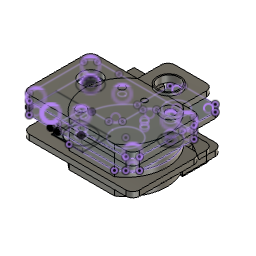
Gearbox v15 (Autodesk Fusion 360 design; units mm, degrees)
Autodesk Fusion 360 part; units mm, degrees
note: some values were not read from the file. Chosen so that the rebuilt part matches the saved one: which face or edge a step refers to; which pieces of a blend or face edit are solid. Set by a fixed rule: which sketch regions a step uses.
sketch "Sketch1" plane through (0, 0, 0) normal (0, 0, 1) x (1, 0, 0) in component "Version 1 Bottom"
  line L0 (5, 5) -> (-6, 5)
  line L1 (-6, 5) -> (-6, -5) construction
  line L2 (-6, -5) -> (5, -5)
  line L3 (6, -4) -> (6, 4)
  line L4 (6, 5) -> (-6, -5) construction
  line L5 (-6, 5) -> (6, -5) construction
  circle A0 centre (3.5799, 2.9833) radius 0.675
  circle A1 centre (-3.5799, -2.9833) radius 0.675
  circle A2 centre (0, 0) radius 1.975
  circle A3 centre (0, 2.735) radius 0.4
  line L6 (0, 1.75) -> (0, 22.5)
  circle A4 centre (-3.2599, 2.7166) radius 0.45
  line L7 (-6, 5) -> (-9.1769, 5)
  line L8 (-10.1769, 4) -> (-10.1769, -4)
  line L9 (-9.1769, -5) -> (-6, -5)
  circle A5 centre (-6.7769, 1.6) radius 0.46
  line L10 (-3.2599, 2.7166) -> (-6.7769, 1.6) construction
  arc A6 (-9.1769, 5) -> (-10.1769, 4) centre (-9.1769, 4) ccw
  arc A7 (-10.1769, -4) -> (-9.1769, -5) centre (-9.1769, -4) ccw
  arc A8 (5, -5) -> (6, -4) centre (5, -4) ccw
  arc A9 (6, 4) -> (5, 5) centre (5, 4) ccw
  circle A10 centre (-6.7769, 1.6) radius 3.4 construction
  circle A11 centre (-3.5799, -2.9833) radius 1.675 construction
  point P0 (-10.1769, -5)
  dimension "d9" = 10
  dimension "d10" = 12
  dimension "d12" = 1.35
  dimension "d13" = 1.35
  dimension "d15" = 3.95
  dimension "d16" = 0.8
  dimension "d18" = 0.9
  dimension "d19" = 3.26
  dimension "d22" = 2.735
  dimension "d27" = 9.32
  dimension "d28" = 4.66
  dimension "d29" = 0.92
  dimension "d31" = 3.69
  dimension "d32" = 1
  dimension "d33" = 1
  dimension "d34" = 1
  dimension "d57" = 6.8
  dimension "d58" = 3.35
  constraint horizontal L0
  constraint perpendicular L0 L1
  constraint parallel L0 L2
  constraint parallel L1 L3
  constraint coincident L4 A2.centre
  constraint coincident L5 A2.centre
  constraint coincident A2.centre origin
  constraint coincident L4 A0.centre
  constraint coincident L4 A1.centre
  constraint coincident A3.centre L6
  constraint coincident L5 A4.centre
  constraint horizontal L7
  constraint vertical L8
  constraint horizontal L9
  constraint collinear L2 L9
  constraint coincident A4.centre L10.start
  constraint coincident A5.centre L10.end
  constraint coincident L1.end L2.start
  constraint tangent L7 A6
  constraint tangent L8 A6
  constraint coincident P0 L8
  constraint coincident P0 L9
  constraint tangent L8 A7
  constraint tangent L9 A7
  constraint equal A6 A7
  constraint coincident L5.end L2
  constraint coincident L5.end L3
  constraint tangent L2 A8
  constraint tangent L3 A8
  constraint coincident L4.start L0
  constraint coincident L4.start L3
  constraint tangent L0 A9
  constraint tangent L3 A9
  constraint concentric A5 A10
  constraint concentric A1 A11
  constraint tangent L0 A10
  constraint tangent L8 A10
  measures "d9" distance of L4.start L5.end
  measures "d10" distance of L4.start L0.end
  measures "d12" diameter of A0
  measures "d13" diameter of A1
  measures "d15" diameter of A2
  measures "d16" diameter of A3
  measures "d18" diameter of A4
  measures "d19" distance of A3.centre A4.centre
  measures "d22" distance of A2.centre A3.centre
  measures "d27" distance of A0.centre A1.centre
  measures "d28" distance of A1.centre A2.centre
  measures "d29" diameter of A5
  measures "d31" distance of A4.centre A5.centre
  measures "d32" radius of A6
  measures "d33" radius of A8
  measures "d34" radius of A9
  measures "d57" diameter of A10
  measures "d58" diameter of A11
extrude "Extrude1" add sketch "Sketch1" along normal blind 0.8 makes body 1 in component "Version 1 Bottom"
ref_plane "WorkPlane1" through (-2.0885, 0, 3.25) normal (0, 0, 1) x (1, 0, 0) in component "Layer2"
sketch "Sketch1 (2)" plane through (0, 0, 3.25) normal (0, 0, 1) x (1, 0, 0) in component "Layer2"
  circle A0 centre (3.5799, 2.9833) radius 0.675
  circle A1 centre (-3.5799, -2.9833) radius 0.675
  line L0 (5, 5) -> (-0.5, 5)
  line L1 (-6, -1) -> (-6, -4)
  line L2 (-5, -5) -> (5, -5)
  line L3 (6, -4) -> (6, 4)
  line L4 (6, 5) -> (-6, -5) construction
  line L5 (-6, 5) -> (6, -5) construction
  circle A2 centre (0, 2.735) radius 0.4
  line L6 (-6, 5) -> (-1.5, 5)
  line L7 (-1.5, 4) -> (-1.5, 1)
  line L8 (-2.5, 0) -> (-5, 0)
  line L9 (-6, 0) -> (-6, 5)
  circle A3 centre (-3.5799, -2.9833) radius 0.675
  arc A4 (-6, -4) -> (-5, -5) centre (-5, -4) ccw
  arc A5 (-5, 0) -> (-6, -1) centre (-5, -1) ccw
  arc A6 (-2.5, 0) -> (-1.5, 1) centre (-2.5, 1) ccw
  arc A7 (-0.5, 5) -> (-1.5, 4) centre (-0.5, 4) ccw
  arc A8 (6, 4) -> (5, 5) centre (5, 4) ccw
  arc A9 (5, -5) -> (6, -4) centre (5, -4) ccw
  dimension "d40" = 10
  dimension "d41" = 12
  dimension "d43" = 1.5
  dimension "d44" = 1
  dimension "d45" = 1
  dimension "d46" = 1
  dimension "d47" = 1
  dimension "d48" = 1
  dimension "d49" = 1
  constraint horizontal L0
  constraint perpendicular L0 L1
  constraint parallel L0 L2
  constraint parallel L1 L3
  constraint coincident L4 origin
  constraint coincident L5 origin
  constraint horizontal L6
  constraint vertical L7
  constraint horizontal L8
  constraint vertical L9
  constraint coincident origin L8
  constraint coincident L4.end L2
  constraint coincident L4.end L1
  constraint tangent L2 A4
  constraint tangent L1 A4
  constraint coincident L9.start L8
  constraint coincident L5.start L1
  constraint tangent L8 A5
  constraint tangent L1 A5
  constraint tangent L7 A6
  constraint tangent L8 A6
  constraint coincident L6.end L7
  constraint coincident L5.start L0
  constraint tangent L7 A7
  constraint tangent L0 A7
  constraint coincident L4.start L3
  constraint coincident L4.start L0
  constraint tangent L3 A8
  constraint tangent L0 A8
  constraint coincident L5.end L3
  constraint coincident L5.end L2
  constraint tangent L3 A9
  constraint tangent L2 A9
  measures "d40" distance of L4.start L5.end
  measures "d41" distance of L1 L3
  measures "d43" distance of A2.centre L7
  measures "d44" radius of A4
  measures "d45" radius of A5
  measures "d46" radius of A6
  measures "d47" radius of A7
  measures "d48" radius of A8
  measures "d49" radius of A9
extrude "Extrude1'" add sketch "Sketch1 (2)" along normal blind 0.8 separate body makes body 2 in component "Layer2"
ref_plane "WorkPlane1" through (-2.0885, 0, 5.02) normal (0, 0, 1) x (1, 0, 0) in component "Layer3"
sketch "Sketch1 (3)" plane through (0, 0, 5.02) normal (0, 0, 1) x (1, 0, 0) in component "Layer3"
  circle A0 centre (3.5799, 2.9833) radius 0.675
  circle A1 centre (-3.5799, -2.9833) radius 0.675
  circle A2 centre (-6.7769, 1.6) radius 0.46
  circle A3 centre (-3.2599, 2.7166) radius 0.45
  circle A4 centre (-6.7769, 1.6) radius 1.52
  arc A5 (-9.1769, 5) -> (-10.1769, 4) centre (-9.1769, 4) ccw
  line L0 (-10.1769, 4) -> (-10.1769, -4)
  arc A6 (-10.1769, -4) -> (-9.1769, -5) centre (-9.1769, -4) ccw
  line L1 (-9.1769, -5) -> (-6, -5)
  line L2 (-6, -5) -> (5, -5)
  arc A7 (5, -5) -> (6, -4) centre (5, -4) ccw
  line L3 (6, -4) -> (6, 4)
  arc A8 (6, 4) -> (5, 5) centre (5, 4) ccw
  line L4 (5, 5) -> (-6, 5)
  line L5 (-6, 5) -> (-9.1769, 5)
  dimension "d55" = 3.04
  constraint concentric A2 A4
  measures "d55" diameter of A4
extrude "Extrude1''" add sketch "Sketch1 (3)" along normal blind 0.8 separate body contours A5 L0 A6 L1 L2 A7 L3 A8 L4 L5 makes body 3 in component "Layer3"
sketch "Sketch1 (4)" plane through (0, 0, 3.25) normal (0, 0, -1) x (1, 0, 0) in component "Version 1 Upper"
  circle A0 centre (0, -2.735) radius 0.4
  circle A1 centre (-3.5799, 2.9833) radius 0.675
  circle A2 centre (3.5799, -2.9833) radius 0.675
  line L0 (-5, 0) -> (-2.5, 0)
  arc A3 (-1.5, -1) -> (-2.5, 0) centre (-2.5, -1) ccw
  line L1 (-1.5, -1) -> (-1.5, -4)
  arc A4 (-1.5, -4) -> (-0.5, -5) centre (-0.5, -4) ccw
  line L2 (-0.5, -5) -> (5, -5)
  arc A5 (5, -5) -> (6, -4) centre (5, -4) ccw
  line L3 (6, -4) -> (6, 4)
  arc A6 (6, 4) -> (5, 5) centre (5, 4) ccw
  line L4 (5, 5) -> (-5, 5)
  arc A7 (-5, 5) -> (-6, 4) centre (-5, 4) ccw
  line L5 (-6, 4) -> (-6, 1)
  arc A8 (-6, 1) -> (-5, 0) centre (-5, 1) ccw
  line L6 (-10.1769, -4) -> (-10.1769, 4)
  arc A9 (-9.1769, 5) -> (-10.1769, 4) centre (-9.1769, 4) ccw
  line L7 (-9.1769, 5) -> (-6, 5)
  line L8 (-6, 5) -> (-5, 5)
  line L9 (-5, 0) -> (-10.1769, 0)
  line L10 (-10.1769, 0) -> (-10.1769, 4)
  constraint coincident L7.end L8.start
  constraint coincident L4.end A7.start
  constraint coincident L0.start A8.end
  constraint coincident L6.end A9.end
  constraint midpoint L6 L9.end
sketch "Sketch2" plane through (0, 0, 5.02) normal (0, 0, -1) x (1, 0, 0) in component "Version 1 Upper"
  circle A0 centre (-6.7769, -1.6) radius 1.52
  circle A1 centre (-3.2599, -2.7166) radius 0.45
  circle A2 centre (3.5799, -2.9833) radius 0.675
  circle A3 centre (-3.5799, 2.9833) radius 0.675
  line L0 (-9.1769, -5) -> (5, -5)
  arc A4 (5, -5) -> (6, -4) centre (5, -4) ccw
  line L1 (6, -4) -> (6, 4)
  arc A5 (6, 4) -> (5, 5) centre (5, 4) ccw
  line L2 (5, 5) -> (-9.1769, 5)
  arc A6 (-9.1769, 5) -> (-10.1769, 4) centre (-9.1769, 4) ccw
  line L3 (-10.1769, 4) -> (-10.1769, -4)
  arc A7 (-10.1769, -4) -> (-9.1769, -5) centre (-9.1769, -4) ccw
  circle A8 centre (-3.2599, -2.7166) radius 0.9
  circle A9 centre (-6.7769, -1.6) radius 3.025
  circle A10 centre (-3.2599, -2.7166) radius 0.65
  circle A11 centre (-6.7769, -1.6) radius 1.72
  dimension "d147" = 1.8
  dimension "d148" = 6.05
  dimension "d152" = 0.2
  dimension "d155" = 0.2
  constraint concentric A1 A8
  constraint concentric A0 A9
  constraint concentric A1 A10
  constraint concentric A0 A11
  measures "d147" diameter of A8
  measures "d148" diameter of A9
  measures "d152" distance of A1 A10
  measures "d155" distance of A0 A11
extrude "Extrude1'''" add sketch "Sketch2" against normal blind 0.8 separate body contours L0 A4 L1 A5 L2 A6 L3 A7 | A8 A9 | A8 A9 | A8 A9 | A10 | A11 makes body 4 in component "Version 1 Upper"
extrude "Extrude2" add sketch "Sketch1 (4)" against normal up to surface (1.77 mm away) bodies 4 in component "Version 1 Upper"
sketch "Sketch1 (5)" plane through (0, 0, 0) normal (0, 0, 1) x (1, 0, 0) in component "Calibration"
  circle A0 centre (-3.5799, -2.9833) radius 0.675
  circle A1 centre (-3.2599, 2.7166) radius 0.45
  circle A2 centre (-6.7769, 1.6) radius 0.46
  circle A3 centre (0, 2.735) radius 0.4
  circle A4 centre (3.5799, 2.9833) radius 0.675
  circle A5 centre (0, 0) radius 1.975
  arc A6 (6, 4) -> (5, 5) centre (5, 4) ccw
  line L0 (5, 5) -> (-9.1769, 5)
  arc A7 (-9.1769, 5) -> (-10.1769, 4) centre (-9.1769, 4) ccw
  line L1 (-10.1769, 4) -> (-10.1769, -4)
  arc A8 (-10.1769, -4) -> (-9.1769, -5) centre (-9.1769, -4) ccw
  line L2 (-9.1769, -5) -> (5, -5)
  arc A9 (5, -5) -> (6, -4) centre (5, -4) ccw
  line L3 (6, -4) -> (6, 4)
  circle A10 centre (-6.6616, -1.798) radius 1.52
  circle A11 centre (-6.7769, 1.6) radius 3.4
  dimension "d68" = 3.04
  dimension "d70" = 6.9
  constraint coincident A10.centre A11
  measures "d68" diameter of A10
  measures "d70" distance of A10.centre A5.centre
extrude "Extrude1''''" add sketch "Sketch1 (5)" along normal blind 0.8 separate body contours A1 A6 L0 L1 A8 L2 A9 L3 A10 A11 | A1 A10 A11 | L0 A7 L1 A11 makes body 5 in component "Calibration"
sketch "Sketch1 (6)" plane through (0, 0, 0) normal (0, 0, 1) x (1, 0, 0) in component "Version 2"
  circle A0 centre (0, 0) radius 6
  line L0 (6, 5) -> (-6, 5)
  line L1 (-6, 5) -> (-6, -5) construction
  line L2 (-6, -5) -> (6, -5)
  line L3 (6, -5) -> (6, 5) construction
  line L4 (6, 5) -> (-6, -5) construction
  line L5 (-6, 5) -> (6, -5) construction
  circle A1 centre (0, 0) radius 1.975
  circle A2 centre (3.5799, 2.9833) radius 0.675
  circle A3 centre (-3.5799, -2.9833) radius 0.675
  circle A4 centre (0, 2.735) radius 0.4
  line L6 (0, 1.75) -> (0, 22.5)
  line L7 (-3.3166, 5) -> (3.3166, 5)
  line L8 (-3.3166, 5) -> (3.3166, 5)
  line L9 (3.3166, 5) -> (3.3166, 6.4944)
  line L10 (3.311, 6.5) -> (-3.3116, 6.5)
  line L11 (-3.3166, 6.495) -> (-3.3166, 5)
  arc A5 (3.3166, 6.4944) -> (3.311, 6.5) centre (3.311, 6.4944) ccw
  arc A6 (-3.3116, 6.5) -> (-3.3166, 6.495) centre (-3.3116, 6.495) ccw
  dimension "d73" = 12
  dimension "d74" = 10
  dimension "d75" = 12
  dimension "d76" = 3.95
  dimension "d100" = 1.5
  constraint coincident A0.centre A1.centre
  constraint horizontal L0
  constraint perpendicular L0 L1
  constraint parallel L0 L2
  constraint parallel L1 L3
  constraint coincident L4 A0.centre
  constraint coincident L5 A0.centre
  constraint horizontal L7
  constraint coincident A0 L7.start
  constraint coincident A0 L7.end
  constraint coincident L0 L7.start
  constraint horizontal L8
  constraint vertical L9
  constraint horizontal L10
  constraint vertical L11
  constraint coincident L7.end L8.end
  constraint tangent L9 A5
  constraint tangent L10 A5
  constraint tangent L10 A6
  constraint tangent L11 A6
  measures "d73" diameter of A0
  measures "d74" distance of L0.start L2.end
  measures "d75" distance of L1.end L2.end
  measures "d76" diameter of A1
  measures "d100" distance of L8 L10
extrude "Extrude1'''''" add sketch "Sketch1 (6)" against normal blind 0.8 separate body contours A0 L0 L2 L7 L8 | A0 L0 L6 L7 L8 | A0 L6 L9 L10 A5 | A0 L0 L6 L7 L8 | A0 L6 L10 L11 A6 makes body 6 in component "Version 2"
ref_plane "WorkPlane1" through (0, 0.75, -2.4) normal (0, 0, 1) x (1, 0, 0) in component "Version 2"
sketch "Sketch2 (2)" plane through (0, 0, -2.4) normal (0, 0, 1) x (1, 0, 0) in component "Version 2"
  circle A0 centre (0, 7.42) radius 0.46
  line L0 (0, 1.75) -> (0, 22.5)
  circle A1 centre (0, 2.735) radius 0.4
  circle A2 centre (0, 0) radius 6
  line L1 (-3.3166, 5) -> (3.3166, 5)
  line L2 (-3.3166, 5) -> (3.3166, 5)
  line L3 (3.3166, 5) -> (3.3166, 9.8)
  line L4 (2.3166, 10.8) -> (-2.3166, 10.8)
  line L5 (-3.3166, 9.8) -> (-3.3166, 5)
  arc A3 (-2.3166, 10.8) -> (-3.3166, 9.8) centre (-2.3166, 9.8) ccw
  arc A4 (3.3166, 9.8) -> (2.3166, 10.8) centre (2.3166, 9.8) ccw
  circle A5 centre (0, 7.42) radius 1
  point P0 (3.3166, 10.8)
  point P1 (3.3166, 5)
  dimension "d88" = 0.92
  dimension "d89" = 4.685
  dimension "d90" = 5.8
  dimension "d91" = 1
  dimension "d92" = 1
  dimension "d99" = 2
  constraint coincident A0.centre L0
  constraint horizontal L2
  constraint vertical L3
  constraint horizontal L4
  constraint vertical L5
  constraint coincident L1.start L2.start
  constraint coincident P1 L1.end
  constraint tangent L4 A3
  constraint tangent L5 A3
  constraint coincident P0 L3
  constraint coincident P0 L4
  constraint tangent L3 A4
  constraint tangent L4 A4
  constraint concentric A0 A5
  measures "d88" diameter of A0
  measures "d89" distance of A0.centre A1.centre
  measures "d90" distance of P1 P0
  measures "d91" radius of A3
  measures "d92" radius of A4
  measures "d99" diameter of A5
extrude "Extrude2'" add sketch "Sketch2 (2)" against normal blind 0.8 separate body contours A0 L0 A5 | A0 L0 A5 | L0 A2 L4 L5 A3 A5 | L0 A2 L3 L4 A4 A5 | L0 A2 L1 L2 | L0 A2 L1 L2 makes body 7 in component "Version 2"
extrude "Extrude3" add sketch "Sketch1 (6)" against normal up to surface (2.4 mm away) contours A0 L0 L6 L7 L8 | A0 L6 L9 L10 A5 | A0 L0 L6 L7 L8 | A0 L6 L10 L11 A6 bodies 6 7 in component "Version 2"
ref_plane "WorkPlane2" through (0, 0.75, 1.65) normal (0, 0, -1) x (-1, 0, 0) in component "Version 2"
sketch "Sketch1 (7)" plane through (0, 0, 1.65) normal (0, 0, -1) x (-1, 0, 0) in component "Upper Deck"
  arc A0 (-3.3166, 5) -> (-3.3166, -5) centre (0, 0) ccw
  line L0 (-3.3166, -5) -> (3.3166, -5)
  arc A1 (3.3166, -5) -> (3.3166, 5) centre (0, 0) ccw
  circle A2 centre (0, 0) radius 1.975
  circle A3 centre (3.5799, -2.9833) radius 0.675
  circle A4 centre (-3.5799, 2.9833) radius 0.675
  circle A5 centre (0, 2.735) radius 0.4
  line L1 (-3.3166, 6.4944) -> (-3.3166, 9.8)
  arc A6 (-2.3166, 10.8) -> (-3.3166, 9.8) centre (-2.3166, 9.8) ccw
  line L2 (-2.3166, 10.8) -> (2.3166, 10.8)
  arc A7 (3.3166, 9.8) -> (2.3166, 10.8) centre (2.3166, 9.8) ccw
  line L3 (3.3166, 9.8) -> (3.3166, 6.495)
  circle A8 centre (0, 7.42) radius 0.46
  circle A9 centre (0, 7.42) radius 1.52
  line L4 (3.3166, 5) -> (-3.3166, 5)
  line L5 (3.3166, 6.495) -> (3.3166, 5)
  line L6 (-3.3166, 6.4944) -> (-3.3166, 5)
  dimension "d104" = 3.04
  constraint concentric A8 A9
  constraint coincident L3.end L5.start
  constraint coincident A1.end L4.start
  constraint coincident L1.start L6.start
  constraint coincident A0.start L4.end
  measures "d104" diameter of A9
extrude "Extrude1''''''" add sketch "Sketch1 (7)" against normal blind 0.8 separate body contours A0 L0 A1 L4 | L1 A6 L2 A7 L3 L4 L5 L6 makes body 8 in component "Upper Deck"
sketch "Sketch1 (8)" plane through (0, 0, 0) normal (0, 0, 1) x (1, 0, 0) in component "Lower Part"
  circle A0 centre (0, 0) radius 6
  line L0 (6, -5) -> (6, 5)
  line L1 (-6, 5) -> (6, -5)
  line L2 (-6, -5) -> (6, -5)
  line L3 (6, 5) -> (-6, -5)
  circle A1 centre (-3.5799, -2.9833) radius 0.675
  circle A2 centre (3.5799, 2.9833) radius 0.675
  line L4 (3.311, 6.5) -> (-3.3116, 6.5)
  line L5 (3.3166, 5) -> (3.3166, 6.4944)
  arc A3 (3.3166, 6.4944) -> (3.311, 6.5) centre (3.311, 6.4944) ccw
  arc A4 (-3.3116, 6.5) -> (-3.3166, 6.495) centre (-3.3116, 6.495) ccw
  line L6 (-3.3166, 6.495) -> (-3.3166, 5)
  line L7 (-3.3166, 5) -> (3.3166, 5)
  line L8 (6, 5) -> (-6, 5)
  line L9 (-6, 5) -> (-6, -5)
  circle A5 centre (0, 2.735) radius 0.4
  point P0 (3.311, 6.4944)
  point P1 (-3.3116, 6.495)
  point P2 (0, 2.735)
  point P3 (0, 1.75)
  point P4 (3.5799, 2.9833)
  point P5 (-3.5799, -2.9833)
extrude "Extrude1'''''''" add sketch "Sketch1 (8)" against normal blind 0.8 separate body contours A0 L7 L8 | A0 L4 L5 A3 A4 L6 | A0 L1 L3 A2 L7 L8 | A0 L1 L3 A2 | A0 L1 L3 A1 | A0 L1 L2 L3 A1 makes body 9 in component "Lower Part"
ref_plane "WorkPlane2" through (0, 0, -1.74) normal (0, 0, 1) x (1, 0, 0) in component "Lower Part"
sketch "Sketch2 (3)" plane through (0, 0, -1.74) normal (0, 0, 1) x (-1, 0, 0) in component "Lower Part"
  arc A0 (-3.3166, -6) -> (-2.8166, -6.5) centre (-2.8166, -6) ccw
  arc A1 (2.8166, -6.5) -> (3.3166, -6) centre (2.8166, -6) ccw
  line L0 (2.8166, -6.5) -> (-2.8166, -6.5)
  circle A2 centre (0, -7.42) radius 0.435
  line L1 (3.3166, -5) -> (-3.3166, -5)
  circle A3 centre (0, -6.305) radius 0.46
  circle A4 centre (0, -2.735) radius 0.38
  circle A5 centre (0, -6.305) radius 0.8
  line L2 (0, -1.75) -> (0, -22.5)
  line L3 (3.3166, -5) -> (-3.3166, -5)
  line L4 (-3.3166, -5) -> (-3.3166, -8.5)
  line L5 (-2.3166, -9.5) -> (2.3166, -9.5)
  line L6 (3.3166, -8.5) -> (3.3166, -5)
  arc A6 (2.3166, -9.5) -> (3.3166, -8.5) centre (2.3166, -8.5) ccw
  arc A7 (-3.3166, -8.5) -> (-2.3166, -9.5) centre (-2.3166, -8.5) ccw
  point P0 (3.3166, -9.5)
  dimension "d109" = 0.92
  dimension "d111" = 3.57
  dimension "d112" = 1.6
  dimension "d113" = 4.5
  dimension "d114" = 1
  dimension "d115" = 1
  constraint concentric A3 A5
  constraint coincident A3.centre L2
  constraint horizontal L3
  constraint vertical L4
  constraint horizontal L5
  constraint vertical L6
  constraint coincident L1.start L3.start
  constraint coincident L1.end L3.end
  constraint coincident P0 L5
  constraint coincident P0 L6
  constraint tangent L5 A6
  constraint tangent L6 A6
  constraint tangent L4 A7
  constraint tangent L5 A7
  measures "d109" diameter of A3
  measures "d111" distance of A3.centre A4.centre
  measures "d112" diameter of A5
  measures "d113" distance of L1.start P0
  measures "d114" radius of A6
  measures "d115" radius of A7
extrude "Extrude2''" add sketch "Sketch2 (3)" against normal blind 1.6 separate body contours A0 L0 L1 A5 L2 L3 L4 | A0 L0 A2 A5 L2 L4 L5 A7 | L0 A3 A5 L2 | L0 A2 A3 A5 L2 | A1 L0 L1 A5 L2 L3 L6 | L0 A3 A5 L2 | A2 A5 L2 | A2 A5 L2 | A1 L0 A2 A5 L2 L5 L6 A6 | L0 A2 A3 A5 L2 | A2 A5 L2 | A2 A5 L2 makes body 10 in component "Lower Part"
extrude "Extrude3'" add sketch "Sketch1 (8)" against normal up to surface (1.74 mm away) contours A0 L7 L8 | A0 L4 L5 A3 A4 L6 bodies 9 10 in component "Lower Part"
extrude "Extrude4" cut sketch "Sketch2 (3)" along normal up to surface (1.74 mm away) contours L0 A3 A5 L2 | L0 A2 A3 A5 L2 | L0 A3 L2 | L0 A3 L2 | L0 A3 A5 L2 | A2 A5 L2 | A2 A5 L2 | L0 A3 L2 | L0 A3 L2 | L0 A2 A3 A5 L2 picked at (-0.1534, -7.2818) picked at (-0.0461, -7.0646) bodies 9 in component "Lower Part"
ref_plane "WorkPlane1" through (0, 0.75, 5) normal (0, 0, 1) x (1, 0, 0) in component "Upper Level"
sketch "Sketch1 (9)" plane through (0, 0, 5) normal (0, 0, 1) x (1, 0, 0) in component "Upper Level"
  line L0 (3.3166, 6.4944) -> (3.3166, 8.5)
  arc A0 (3.3166, 8.5) -> (2.3166, 9.5) centre (2.3166, 8.5) ccw
  line L1 (2.3166, 9.5) -> (-2.3166, 9.5)
  arc A1 (-2.3166, 9.5) -> (-3.3166, 8.5) centre (-2.3166, 8.5) ccw
  line L2 (-3.3166, 8.5) -> (-3.3166, 6.495)
  line L3 (-3.3166, 6.495) -> (-3.3166, 5)
  arc A2 (-3.3166, 5) -> (-3.3166, -5) centre (0, 0) ccw
  line L4 (-3.3166, -5) -> (3.3166, -5)
  arc A3 (3.3166, -5) -> (3.3166, 5) centre (0, 0) ccw
  line L5 (3.3166, 5) -> (3.3166, 6.4944)
  circle A4 centre (3.5799, 2.9833) radius 0.675
  circle A5 centre (0, 2.735) radius 0.4
  circle A6 centre (-3.5799, -2.9833) radius 0.675
  circle A7 centre (0, 6.305) radius 1.52
  point P0 (0, 6.305)
  dimension "d126" = 3.04
  constraint coincident P0 A7.centre
  measures "d126" diameter of A7
extrude "Extrude1''''''''" add sketch "Sketch1 (9)" along normal blind 0.8 separate body makes body 11 in component "Upper Level"
sketch "Sketch5" plane through (3.3166, 0, 0) normal (1, 0, 0) x (0, 1, 0) in component "Version 2"
  line L0 (6.4944, 0) -> (5, 0)
  line L1 (5, 0) -> (5, -0.8)
  line L2 (5, -0.8) -> (5, -3.2)
  line L3 (5, -3.2) -> (9.8, -3.2)
  line L4 (9.8, -3.2) -> (9.8, -2.4)
  line L5 (9.8, -2.4) -> (6.4944, -2.4)
  line L6 (6.4944, -2.4) -> (6.4944, 0)
  line L7 (6.4944, 0) -> (7.42, -2.4)
  line L8 (6.4944, -2.4) -> (6.4944, 0)
  point P0 (7.42, -2.4)
  constraint coincident L0.start L6.end
  constraint coincident P0 L7.end
  constraint coincident L5.end L6.start
extrude "Extrude6" add sketch "Sketch5" against normal up to surface (6.6332 mm away) contours L5 L6 L7 L8 bodies 6 in component "Version 2"
extrude "Extrude7" cut sketch "Sketch2 (2)" along normal up to surface (2.4 mm away) contours A0 L0 | A0 L0 A5 | A0 L0 | A0 L0 A5 bodies 6 in component "Version 2"
sketch "Sketch2 (4)" plane through (0, 0, 5.8) normal (0, 0, 1) x (-1, 0, 0) in component "Upper Level"
  circle A0 centre (0, -6.305) radius 1.52
  circle A1 centre (-3.5799, -2.9833) radius 0.675
  circle A2 centre (0, -2.735) radius 0.4
  circle A3 centre (3.5799, 2.9833) radius 0.675
  line L0 (-3.3166, -5) -> (-3.3166, -8.5)
  arc A4 (-3.3166, -8.5) -> (-2.3166, -9.5) centre (-2.3166, -8.5) ccw
  line L1 (-2.3166, -9.5) -> (2.3166, -9.5)
  arc A5 (2.3166, -9.5) -> (3.3166, -8.5) centre (2.3166, -8.5) ccw
  line L2 (3.3166, -8.5) -> (3.3166, -5)
  arc A6 (3.3166, -5) -> (3.3166, 5) centre (0, 0) ccw
  line L3 (3.3166, 5) -> (-3.3166, 5)
  arc A7 (-3.3166, 5) -> (-3.3166, -5) centre (0, 0) ccw
  circle A8 centre (0, -6.305) radius 1.52
  circle A9 centre (0, -6.305) radius 1.72
  dimension "d140" = 0.2
  constraint concentric A8 A9
  measures "d140" distance of A8 A9
extrude "Extrude2'''" add sketch "Sketch2 (4)" along normal blind 0.4 contours A9 bodies 11 in component "Upper Level"
sketch "Sketch3" plane through (0, 0, 5) normal (0, 0, -1) x (1, 0, 0) in component "Upper Level"
  circle A0 centre (0, -6.305) radius 1.52
  circle A1 centre (3.5799, -2.9833) radius 0.675
  circle A2 centre (0, -2.735) radius 0.4
  circle A3 centre (-3.5799, 2.9833) radius 0.675
  line L0 (3.3166, -8.5) -> (3.3166, -5)
  arc A4 (3.3166, -5) -> (3.3166, 5) centre (0, 0) ccw
  line L1 (3.3166, 5) -> (-3.3166, 5)
  arc A5 (-3.3166, 5) -> (-3.3166, -5) centre (0, 0) ccw
  line L2 (-3.3166, -5) -> (-3.3166, -8.5)
  arc A6 (-3.3166, -8.5) -> (-2.3166, -9.5) centre (-2.3166, -8.5) ccw
  line L3 (-2.3166, -9.5) -> (2.3166, -9.5)
  arc A7 (2.3166, -9.5) -> (3.3166, -8.5) centre (2.3166, -8.5) ccw
  circle A8 centre (0, -6.305) radius 3.025
  point P0 (0, -6.305)
  dimension "d143" = 6.05
  constraint coincident P0 A0.centre
  measures "d143" diameter of A8
extrude "Extrude3''" cut sketch "Sketch3" against normal blind 0.2 contours A8 bodies 11 in component "Upper Level"
extrude "Extrude3'''" cut sketch "Sketch2" along normal through all contours A8 A9 | A11 picked at (-4.6148, -2.9553) bodies 4 in component "Version 1 Upper"
extrude "Extrude4'" add sketch "Sketch2" along normal blind 0.2 contours A10 bodies 4 in component "Version 1 Upper"
extrude "Extrude5" add sketch "Sketch2" along normal blind 0.2 contours A11 bodies 4 in component "Version 1 Upper"
extrude "Extrude6'" cut sketch "Sketch1 (4)" against normal up to surface (2.57 mm away) contours A0 bodies 4 in component "Version 1 Upper"
fillet "Fillet3" radius 1 3 edges at (-4.2097, 0, 4.135) (-9.3442, 0, 4.135) (-10.1769, 0, 4.135) on bodies 4 in component "Version 1 Upper"
sketch "Sketch2 (5)" plane through (0, 0, 1.65) normal (0, 0, -1) x (1, 0, 0) in component "Upper Deck"
  circle A0 centre (0, -7.42) radius 1.52
  circle A1 centre (0, 0) radius 1.975
  circle A2 centre (0, -2.735) radius 0.4
  circle A3 centre (-3.5799, 2.9833) radius 0.675
  circle A4 centre (3.5799, -2.9833) radius 0.675
  arc A5 (2.3166, -10.8) -> (3.3166, -9.8) centre (2.3166, -9.8) ccw
  line L0 (3.3166, -9.8) -> (3.3166, -5)
  arc A6 (3.3166, -5) -> (3.3166, 5) centre (0, 0) ccw
  line L1 (3.3166, 5) -> (-3.3166, 5)
  arc A7 (-3.3166, 5) -> (-3.3166, -5) centre (0, 0) ccw
  line L2 (-3.3166, -5) -> (-3.3166, -9.8)
  arc A8 (-3.3166, -9.8) -> (-2.3166, -10.8) centre (-2.3166, -9.8) ccw
  line L3 (-2.3166, -10.8) -> (2.3166, -10.8)
  circle A9 centre (0, -7.42) radius 2.52
  dimension "d166" = 1
  constraint concentric A0 A9
  measures "d166" distance of A0 A9
extrude "Extrude3''''" add sketch "Sketch2 (5)" along normal blind 0.8 contours A9 bodies 8 in component "Upper Deck"
sketch "Sketch1 (10)" plane through (0, 0, 2.45) normal (0, 0, 1) x (-1, 0, 0) in component "Distancers"
  circle A0 centre (0, -7.42) radius 1.52
  circle A1 centre (0, 0) radius 1.975
  circle A2 centre (0, -2.735) radius 0.4
  circle A3 centre (3.5799, 2.9833) radius 0.675
  circle A4 centre (-3.5799, -2.9833) radius 0.675
  arc A5 (-3.3166, -9.8) -> (-2.3166, -10.8) centre (-2.3166, -9.8) ccw
  line L0 (-2.3166, -10.8) -> (2.3166, -10.8)
  arc A6 (2.3166, -10.8) -> (3.3166, -9.8) centre (2.3166, -9.8) ccw
  line L1 (3.3166, -9.8) -> (3.3166, -5)
  arc A7 (3.3166, -5) -> (3.3166, 5) centre (0, 0) ccw
  line L2 (3.3166, 5) -> (-3.3166, 5)
  arc A8 (-3.3166, 5) -> (-3.3166, -5) centre (0, 0) ccw
  line L3 (-3.3166, -5) -> (-3.3166, -9.8)
  circle A9 centre (0, 0) radius 3.275
  line L4 (-2.2799, -2.3511) -> (-2.2799, -3.9633)
  line L5 (-2.2799, -3.9633) -> (-3.3166, -5)
  line L6 (0, -2.5) -> (0, -20)
  line L7 (2.2799, -2.3511) -> (2.2799, -3.9633)
  line L8 (2.2799, -3.9633) -> (3.3166, -5)
  dimension "d169" = 1.3
  dimension "d170" = 1.3
  dimension "d171" = 135
  constraint coincident A9 L4.start
  constraint vertical L4
  constraint coincident A8.end L3.start
  constraint symmetric L4.start L6 L7.start
  constraint symmetric L4.end L6 L7.end
  constraint symmetric A8.end L6 L1.end
  measures "d170" distance of A4.centre L4
  measures "d171" angle of L4 L5
extrude "Extrude1'''''''''" add sketch "Sketch1 (10)" along normal blind 2.2 separate body contours A7 L2 A8 A9 L4 L5 L7 L8 makes body 12 in component "Distancers"
sketch "Sketch1 (11)" plane through (0, 0, 2.45) normal (0, 0, 1) x (-1, 0, 0) in component "Distancer"
  circle A0 centre (0, -7.42) radius 1.52
  circle A1 centre (0, 0) radius 1.975
  circle A2 centre (0, -2.735) radius 0.4
  circle A3 centre (3.5799, 2.9833) radius 0.675
  circle A4 centre (-3.5799, -2.9833) radius 0.675
  arc A5 (-3.3166, -9.8) -> (-2.3166, -10.8) centre (-2.3166, -9.8) ccw
  line L0 (-2.3166, -10.8) -> (2.3166, -10.8)
  arc A6 (2.3166, -10.8) -> (3.3166, -9.8) centre (2.3166, -9.8) ccw
  line L1 (3.3166, -9.8) -> (3.3166, -5)
  arc A7 (3.3166, -5) -> (3.3166, 5) centre (0, 0) ccw
  line L2 (3.3166, 5) -> (-3.3166, 5)
  arc A8 (-3.3166, 5) -> (-3.3166, -5) centre (0, 0) ccw
  line L3 (-3.3166, -5) -> (-3.3166, -9.8)
  circle A9 centre (-3.5799, -2.9833) radius 1.34
  line L4 (1.3299, 0.9833) -> (5.8299, 0.9833)
  line L5 (5.8299, 0.9833) -> (5.8299, 4.9833)
  line L6 (5.8299, 4.9833) -> (1.3299, 4.9833)
  line L7 (1.3299, 4.9833) -> (1.3299, 0.9833)
  line L8 (1.3299, 0.9833) -> (5.8299, 4.9833) construction
  line L9 (5.8299, 0.9833) -> (1.3299, 4.9833) construction
  circle A10 centre (3.5799, 2.9833) radius 1.875
  point P0 (3.5799, 2.9833)
  dimension "d174" = 4
  dimension "d175" = 4.5
  dimension "d180" = 1.2
  constraint concentric A4 A9
  constraint tangent A8 A9
  constraint horizontal L4
  constraint perpendicular L4 L5
  constraint parallel L4 L6
  constraint parallel L5 L7
  constraint coincident L8 P0
  constraint coincident L9 P0
  constraint coincident P0 A3.centre
  measures "d174" distance of L4.start L6.end
  measures "d175" distance of L5 L7
  measures "d180" distance of A3 A10
extrude "Extrude1''''''''''" add sketch "Sketch1 (11)" along normal blind 3.5 separate body contours A9 makes body 13 in component "Distancer"
extrude "Extrude2''''" add sketch "Sketch1 (11)" along normal blind 2.5 separate body contours A1 L4 L7 | A1 A7 L4 L5 L6 L7 A10 | A7 L5 L6 A10 | A7 A10 | A7 A10 picked at (1.4686, 1.151) makes body 14 in component "Distancer"
move_body "Move1" bodies 14 to x (1, 0, 0) y (0, 1, 0) z (0, 0, 1) at (0, 8, 0) in component "Distancer"
extrude "Extrude3'''''" add sketch "Sketch1 (11)" along normal blind 2.5 separate body contours A7 A10 | A7 A10 makes body 15 in component "Distancer"
component "Version 1 Bottom" placed x (1, 0, 0) y (0, 1, 0) z (0, 0, 1) at (0, 0, 0)
component "Layer2" placed x (1, 0, 0) y (0, 1, 0) z (0, 0, 1) at (0, 0, 0)
component "Layer3" placed x (1, 0, 0) y (0, 1, 0) z (0, 0, 1) at (0, 0, 0)
component "Version 1 Upper" placed x (1, 0, 0) y (0, 1, 0) z (0, 0, 1) at (0, 0, 0)
component "Calibration" placed x (1, 0, 0) y (0, 1, 0) z (0, 0, 1) at (0, 0, 0)
component "Version 2" placed x (1, 0, 0) y (0, 1, 0) z (0, 0, 1) at (0, 0, 0)
component "Version 3" placed x (1, 0, 0) y (0, 1, 0) z (0, 0, 1) at (0, 0, 0)
component "Distancers" placed x (1, 0, 0) y (0, 1, 0) z (0, 0, 1) at (0, 0, 0)
component "Distancer" placed x (1, 0, 0) y (0, 1, 0) z (0, 0, 1) at (0, 0, 0)
component "Upper Deck" placed x (1, 0, 0) y (0, 1, 0) z (0, 0, 1) at (0, 0, 0) in component "Version 2"
component "Lower Part" placed x (1, 0, 0) y (0, 1, 0) z (0, 0, 1) at (0, 0, 0) in component "Version 3"
component "Upper Level" placed x (1, 0, 0) y (0, 1, 0) z (0, 0, 1) at (0, 0, 0) in component "Version 3"
equation "motor_gear_hole_diam = 3.95 mm"
equation "screw_diam = 1.35 mm"
equation "width = 12 mm"
equation "height = 10 mm"
equation "screw_distance = 9.32 mm"
equation "shaft2_diam = 0.85 mm + tolerance"
equation "shaft1_diam = 0.75 mm + tolerance"
equation "shaft3_diam = 0.87 mm + tolerance"
equation "d9 = height"
equation "d10 = width"
equation "d12 = screw_diam"
equation "d13 = screw_diam"
equation "d15 = motor_gear_hole_diam"
equation "d16 = shaft1_diam"
equation "d18 = shaft2_diam"
equation "d19 = distance1_2"
equation "distance1_2 = 3.25 mm + distance_buffer"
equation "distance2_3 = 3.68 mm + distance_buffer"
equation "d22 = distance0_1"
equation "distance0_1 = 2.725 mm + distance_buffer"
equation "extension_length = 5 mm"
equation "d27 = screw_distance"
equation "d28 = screw_distance / 2"
equation "d29 = shaft3_diam"
equation "d31 = distance2_3"
equation "plate_thickness = 0.8 mm"
equation "d36 = plate_thickness"
equation "layer0_1_distance = 2.45 mm"
equation "d39 = layer0_1_distance"
equation "d40 = height"
equation "d41 = width"
equation "d44 = radius"
equation "d45 = radius"
equation "d46 = radius"
equation "d47 = radius"
equation "d48 = radius"
equation "d49 = radius"
equation "radius = 1.00 mm"
equation "d51 = plate_thickness"
equation "layer0_2_distance = layer0_1_distance + 1.77 mm"
equation "d54 = layer0_2_distance"
equation "d55 = output_shaft_diam"
equation "d58 = screw_diam + 2 mm"
equation "d59 = plate_thickness"
equation "d61 = -plate_thickness"
equation "d68 = output_shaft_diam"
equation "output_shaft_diam = 2.99 mm + tolerance"
equation "d71 = plate_thickness"
equation "d76 = motor_gear_hole_diam"
equation "distance1_3 = 4.675 mm + distance_buffer"
equation "d84 = -plate_thickness"
equation "lowest_gear_ratio_offset = 2.4 mm"
equation "d87 = -lowest_gear_ratio_offset"
equation "d88 = shaft3_diam"
equation "d89 = distance1_3"
equation "d93 = -plate_thickness"
equation "d101 = -layer0_1_distance"
equation "d102 = -plate_thickness"
equation "d104 = output_shaft_diam"
equation "tolerance = 0.05 mm"
equation "distance_buffer = 0.01 mm"
equation "d107 = -plate_thickness"
equation "d109 = shaft3_diam"
equation "distance1_3_small = 3.57 mm"
equation "d111 = distance1_3_small"
equation "d116 = -plate_thickness * 2"
equation "d123 = -lowest_gear_ratio_offset_small"
equation "lowest_gear_ratio_offset_small = lowest_gear_ratio_offset - 0.66 mm"
equation "d126 = output_shaft_diam"
equation "d127 = plate_thickness"
equation "d164 = radius"
